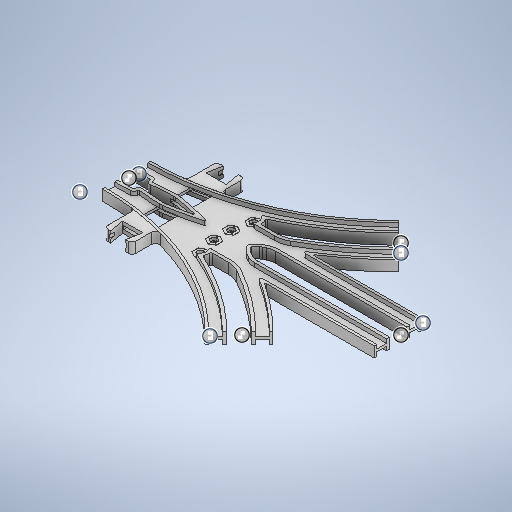
# Autodesk Inventor part: RR_SingleTurnout-all
Saved by Autodesk Inventor 2025.1 (Build 291241000, 241)
## iProperties
Created: 2025-03-05
Part Number: RR_SingleTurnout-all
Material: 一般
Document SubType Name: Modeling
Designer: kumagai
Density: 1 g/cm^3
Appearance: 既定
d0: 244.000 mm
d1: 10.000 mm
d2: 215.000 mm
d3: 5.000 mm
d4: 38.000 mm
d5: 18.600 mm
d6: 2.000 mm
d7: 2.400 mm
d8: 215.000 mm
d9: 45.00 deg
d11: 15.000 mm
d12: 15.000 mm
d13: 2.000 mm
d14: 0.00 deg
d15: 8.400 mm
d16: 0.00 deg
d17: 0.500 mm
d18: 1.000 mm
d19: 20.000 mm
d20: 15.000 mm
d23: 2.500 mm
d30: 5.000 mm
d32: 4.000 mm
d33: 3.000 mm
d34: 4.500 mm
d35: 2.400 mm
d36: 4.000 mm
d37: 1.000 mm
d38: 5.000 mm
d39: 19.000 mm
d41: 0.000 mm
d42: 0.000 mm
d43: 0.000 mm
d44: 0.000 mm
d45: 0.000 mm
d46: 0.000 mm
d47: 0.000 mm
d48: 0.000 mm
d49: 0.000 mm
d51: 5.000 mm
d52: 10.200 mm
d53: 0.300 mm
d55: 2.400 mm
d56: 10.000 mm
d57: 8.000 mm
d58: 0.300 mm
d59: 2.000 mm
d60: 5.000 mm
d62: 2.400 mm
d63: 1.200 mm
d65: 1.200 mm
d66: 42.200 mm
d67: 45.800 mm
TurnoutRadius: 215.000 mm
d40: 19.000 mm
d50: 10.200 mm
PrinterOffset: 0.000 mm
StraightLength: 215.000 mm
RailWidth: 38.000 mm
OuterWall: 2.000 mm
InnerWall: 2.400 mm
InsideWidth: 18.600 mm
RailHeight: 8.400 mm
RailDepth: 3.200 mm
ConnectorLength: 15.000 mm
JointMW1: 13.000 mm
JointMW2: 9.400 mm
JointMH: 9.000 mm
JointFW1: 13.300 mm
JointFW2: 9.600 mm
JointFH: 9.500 mm
DoubleWidth: 60.000 mm
ViaductHeight: 66.000 mm
SupportGap: 0.200 mm
SupportRib: 0.650 mm
JointRadius: 12.000 mm
JointRSLength: 15.000 mm
JointRSTP: 3.000 mm
RailThick: 2.000 mm
d100: 34.048 mm
d126: 0.081 mm
d174: -0.352 mm
d175: 0.482 mm
d178: 0.336 mm
d179: 0.374 mm
Author: kumagai
Autodesk Inventor part; units mm, degrees
ref_plane "YZ Plane" through (0, 0, 0) normal (1, 0, 0) x (0, 1, 0)
sketch "MainSketch" plane through (0, 0, 0) normal (0, 1, 0) x (-1, 0, 0)
  line L0 (0, -344.2613) -> (0, 286.2613) projected
  line L1 (-272.9287, 0) -> (62.5724, 0) projected
  line L2 (14.6437, -29) -> (-5, -29)
  line L3 (-5, -49.5106) -> (-5, -5.6416)
  line L4 (-5, -48) -> (0, -48)
  line L5 (-5, -10) -> (0, -10)
  line L6 (-5, -38.3) -> (0, -38.3)
  line L7 (-5, -19.7) -> (0, -19.7)
  line L8 (-5, -46) -> (0, -46)
  line L9 (-5, -35.9) -> (0, -35.9)
  line L10 (-5, -22.1) -> (0, -22.1)
  line L11 (-5, -12) -> (0, -12)
  line L12 (-10, -10) -> (-10, -29)
  line L13 (-225, -48) -> (-225, -29)
  line L14 (-120.9077, -19.7) -> (-225, -19.7)
  arc A0 (-10, -48) -> (-148.5929, -105.4071) centre (-10, -244) ccw
  arc A1 (-10, -46) -> (-150.0071, -103.9929) centre (-10, -244) ccw
  line L15 (-143.2215, -110.7785) -> (-189.5102, -64.4898)
  line L16 (-210, -35.9) -> (-210, -29)
  line L17 (-146.1596, -86.6272) -> (-155.9415, -76.8453)
  arc A2 (-133.8847, -47.8455) -> (-174.0488, -79.9512) centre (-10, -244) ccw
  arc A3 (-139.2229, -48.9168) -> (-175.463, -78.537) centre (-10, -244) ccw
  line L18 (-139.499, -48) -> (-225, -48)
  line L19 (-134.4186, -46) -> (-225, -46)
  arc A4 (-118.9103, -50.6657) -> (-166.907, -87.093) centre (-10, -244) ccw
  arc A5 (-120.0882, -48.5746) -> (-168.6041, -85.3959) centre (-10, -244) ccw
  line L20 (-94.2219, -46) -> (-110.2721, -46)
  arc A6 (-111.9271, -35.5897) -> (-114.1724, -36.7028) centre (-10, -244) ccw
  line L21 (-120.9077, -35.9) -> (-225, -35.9)
  line L22 (-120.9077, -38.3) -> (-225, -38.3)
  arc A7 (-133.8847, -47.8455) -> (-134.4186, -46) centre (-134.4186, -47) ccw
  arc A8 (-139.2229, -48.9168) -> (-139.499, -48) centre (-139.499, -48.5) ccw
  arc A9 (-110.2721, -48.4) -> (-118.9103, -50.6657) centre (-110.2721, -66) ccw
  arc A10 (-110.2721, -46) -> (-120.0882, -48.5746) centre (-110.2721, -66) ccw
  arc A11 (-120.9077, -38.3) -> (-114.1724, -36.7028) centre (-120.9077, -23.3) ccw
  arc A12 (-120.9077, -35.9) -> (-115.25, -34.5584) centre (-120.9077, -23.3) ccw
  arc A13 (-143.5264, -51.2283) -> (-148.5252, -54.7884) centre (-10, -244) ccw
  arc A14 (-112.9815, -33.4337) -> (-115.25, -34.5584) centre (-10, -244) ccw
  line L23 (-120.9077, -22.1) -> (-225, -22.1)
  circle A15 centre (-86.125, -22.2) radius 2.5
  arc A16 (-96.415, -52.9331) -> (-105.3417, -57.2273) centre (-10, -244) ccw
  arc A17 (-96.4922, -49.4759) -> (-95.7188, -53.2122) centre (-89.6121, -50) ccw
  arc A18 (-93.3838, -47.5455) -> (-92.1285, -53.7307) centre (-89.6121, -50) ccw
  arc A19 (-96.1897, -54.5879) -> (-157.1489, -96.8511) centre (-10, -244) ccw
  line L24 (-97.4893, -48.4) -> (-110.2721, -48.4)
  arc A20 (-92.2877, -55.4762) -> (-155.4519, -98.5481) centre (-10, -244) ccw
  arc A21 (-92.2877, -55.4762) -> (-92.1285, -53.7307) centre (-92.6877, -54.5597) ccw
  arc A22 (-93.3838, -47.5455) -> (-94.2219, -46) centre (-94.2219, -47) ccw
  arc A23 (-96.1897, -54.5879) -> (-95.7188, -53.2122) centre (-96.6039, -53.6777) ccw
  arc A24 (-96.4922, -49.4759) -> (-97.4893, -48.4) centre (-97.4893, -49.4) ccw
  circle A25 centre (-89.6121, -50) radius 2.5
  line L25 (-42.4799, -17.7596) -> (-25.8571, -19.9879)
  arc A26 (-25.9153, -20.5847) -> (-85.6348, -24.6515) centre (-40.1446, -252.1479) ccw
  arc A27 (-85.7928, -19.7222) -> (-85.6348, -24.6515) centre (-86.125, -22.2) ccw
  arc A28 (-25.9153, -20.5847) -> (-25.8571, -19.9879) centre (-25.8969, -20.2853) ccw
  arc A29 (-42.4799, -17.7596) -> (-76.3848, -20.5664) centre (-40.1446, -252.1479) ccw
  line L26 (-85.7928, -19.7222) -> (-79.2595, -20.598)
  arc A30 (-79.2595, -20.598) -> (-76.3848, -20.5664) centre (-77.9308, -10.6866) ccw
  circle A31 centre (-89.6121, -50) radius 4
  line L27 (-89.754, -46.0025) -> (-25.5965, -43.7259)
  arc A32 (-25.552, -44.3238) -> (-40.8225, -46.6677) centre (-3.1703, -241.0547) ccw
  arc A33 (-25.552, -44.3238) -> (-25.5965, -43.7259) centre (-25.5859, -44.0257) ccw
  arc A34 (-74.4895, -48.1141) -> (-87.9633, -53.6443) centre (-3.1703, -241.0547) ccw
  line L28 (-72.9332, -47.8071) -> (-40.8225, -46.6677)
  arc A35 (-72.9332, -47.8071) -> (-74.4895, -48.1141) centre (-72.7559, -52.804) ccw
  arc A36 (-44.0479, -18.9806) -> (-84.6326, -23.2308) centre (-40.1446, -252.1479) ccw
  arc A37 (-27.9859, -39.0878) -> (-44.4613, -41.2072) centre (-10, -244) ccw
  line L29 (-31.1334, -19.7) -> (-47.6548, -19.7)
  arc A38 (-10, -22.1) -> (-22.0271, -22.4262) centre (-10, -244) ccw
  arc A39 (-44.7432, -24.8368) -> (-62.9678, -28.5145) centre (-10, -244) ccw
  arc A40 (-10, -19.7) -> (-22.1572, -20.0297) centre (-10, -244) ccw
  arc A41 (-45.119, -22.4664) -> (-72.2793, -28.5197) centre (-10, -244) ccw
  arc A42 (-25.457, -23.6967) -> (-43.178, -22.3501) centre (-51.8841, -254.1867) ccw
  line L30 (-24.9, -22.9254) -> (-24.9, -23.2)
  arc A43 (-25.457, -23.6967) -> (-24.9, -23.2) centre (-25.4, -23.2) ccw
  arc A44 (-22.1572, -20.0297) -> (-24.9, -22.9254) centre (-22, -22.9254) ccw
  arc A45 (-43.178, -22.3501) -> (-45.119, -22.4664) centre (-43.5532, -32.343) ccw
  arc A46 (-25.7303, -26.0811) -> (-43.268, -24.7484) centre (-51.8841, -254.1867) ccw
  arc A47 (-22.0271, -22.4262) -> (-22.5, -22.9254) centre (-22, -22.9254) ccw
  line L31 (-22.5, -22.9254) -> (-22.5, -23.2)
  arc A48 (-25.7303, -26.0811) -> (-22.5, -23.2) centre (-25.4, -23.2) ccw
  arc A49 (-43.268, -24.7484) -> (-44.7432, -24.8368) centre (-43.5532, -32.343) ccw
  line L32 (-55.2, -53.283) -> (-55.2, -10)
  line L33 (-40.8, -50.4351) -> (-40.8, -10)
  line L34 (-48, 3.552) -> (-48, 5.2256)
  line L35 (-59, -61.5) -> (-37, -61.5)
  line L36 (-40.8, -10) -> (-40.8, -7.4996)
  line L37 (-55.2, -10) -> (-55.2, -7.4996)
  line L38 (-48, -61.9179) -> (-48, -64.1825)
  line L39 (-37, -61.5) -> (-37, -70.5)
  line L40 (-40, -73.5) -> (-42, -73.5)
  line L41 (-42, -73.5) -> (-40, -62)
  line L42 (-40, -62) -> (-56, -62)
  line L43 (-56, -62) -> (-54, -73.5)
  line L44 (-54, -73.5) -> (-56, -73.5)
  line L45 (-59, -70.5) -> (-59, -58.1371)
  arc A50 (-40, -73.5) -> (-37, -70.5) centre (-40, -70.5) ccw
  arc A51 (-59, -70.5) -> (-56, -73.5) centre (-56, -70.5) ccw
  line L46 (-37, -61.5) -> (-37, -49.8686)
  line L47 (-40.8, -50.4351) -> (-40.8, -62)
  line L48 (-55.2, -53.283) -> (-55.2, -62)
  arc A52 (-34.3731, -49.5213) -> (-37, -52.498) centre (-34, -52.498) ccw
  arc A53 (-59, -58.1371) -> (-62.8083, -55.2481) centre (-62, -58.1371) ccw
  line L49 (-10, -29) -> (-225, -29)
  arc A54 (-151.7465, 120.5538) -> (-11.4945, 29.8813) centre (-10, 186) ccw
  arc A55 (-22.0271, -35.5738) -> (-10, -35.9) centre (-10, 186) ccw
  arc A56 (-62.9678, -29.4855) -> (-44.7432, -33.1632) centre (-10, 186) ccw
  arc A57 (-22.1572, -37.9703) -> (-10, -38.3) centre (-10, 186) ccw
  arc A58 (-72.2793, -29.4803) -> (-45.119, -35.5336) centre (-10, 186) ccw
  arc A59 (-43.178, -35.6499) -> (-25.457, -34.3033) centre (-51.8841, 196.1867) ccw
  arc A60 (-43.268, -33.2516) -> (-25.7303, -31.9189) centre (-51.8841, 196.1867) ccw
  arc A61 (-45.119, -35.5336) -> (-43.178, -35.6499) centre (-43.5532, -25.657) ccw
  arc A62 (-44.7432, -33.1632) -> (-43.268, -33.2516) centre (-43.5532, -25.657) ccw
  line L50 (-24.9, -35.0746) -> (-24.9, -34.8)
  arc A63 (-24.9, -35.0746) -> (-22.1572, -37.9703) centre (-22, -35.0746) ccw
  arc A64 (-22.5, -35.0746) -> (-22.0271, -35.5738) centre (-22, -35.0746) ccw
  line L51 (-22.5, -35.0746) -> (-22.5, -34.8)
  arc A65 (-24.9, -34.8) -> (-25.457, -34.3033) centre (-25.4, -34.8) ccw
  arc A66 (-22.5, -34.8) -> (-25.7303, -31.9189) centre (-25.4, -34.8) ccw
  arc A67 (-62.9678, -28.5145) -> (-63.3485, -29) centre (-62.8485, -29) ccw
  arc A68 (-72.2793, -28.5197) -> (-72.6405, -29) centre (-72.1405, -29) ccw
  arc A69 (-108.1902, -15.666) -> (-89.3785, -23.7845) centre (-10, 186) ccw
  arc A70 (-91.0057, 5.3288) -> (-16.6975, -11.8867) centre (-10, 186) ccw
  arc A71 (-122.8924, 131.193) -> (-43.8763, 65.1658) centre (-10, 186) ccw
  arc A72 (-148.5252, -3.2116) -> (-143.5264, -6.7717) centre (-10, 186) ccw
  circle A73 centre (-86.125, -35.8) radius 2.5
  arc A74 (-85.7286, -33.3316) -> (-25.8975, -35.1189) centre (-48.9436, 195.7336) ccw
  line L52 (-25.8166, -35.7131) -> (-42.3424, -38.5735)
  arc A75 (-25.8166, -35.7131) -> (-25.8975, -35.1189) centre (-25.8677, -35.4174) ccw
  line L53 (-85.6986, -38.2634) -> (-79.2034, -37.1391)
  arc A76 (-76.3296, -37.0611) -> (-79.2034, -37.1391) centre (-77.4979, -46.9926) ccw
  arc A77 (-76.3296, -37.0611) -> (-42.3424, -38.5735) centre (-48.9436, 195.7336) ccw
  arc A78 (-49.1227, -37.4664) -> (-46.0444, -37.4484) centre (-48.9436, 195.7336) ccw
  line L54 (-86.4807, -38.2746) -> (-94.1197, -37.1765)
  arc A79 (-94.2268, -36.2144) -> (-94.1197, -37.1765) centre (-94.0486, -36.6816) ccw
  line L55 (-87.0159, -33.4641) -> (-94.2268, -36.2144)
  line L56 (-76.4926, -34.8148) -> (-77.6457, -34.6296)
  arc A80 (-96.055, -36.8647) -> (-107.6082, -42.0517) centre (-10, -244) ccw
  circle A81 centre (-89.6121, -8) radius 4
  line L57 (-89.6178, -12) -> (-25.42, -12.0915)
  arc A82 (-88.0883, -4.3016) -> (-74.4341, -9.37) centre (-9.7235, 185.8863) ccw
  arc A83 (-74.4341, -9.37) -> (-72.8683, -9.6239) centre (-72.8611, -4.6239) ccw
  line L58 (-72.8683, -9.6239) -> (-40.7373, -9.6697)
  arc A84 (-40.7373, -9.6697) -> (-25.3959, -11.4925) centre (-9.7235, 185.8863) ccw
  arc A85 (-25.42, -12.0915) -> (-25.3959, -11.4925) centre (-25.4196, -11.7915) ccw
  line L59 (-41.4, -73.5) -> (-41.4, -70.05)
  line L60 (-54.6, -73.5) -> (-54.6, -70.05)
  line L61 (-21.7393, -64.7371) -> (-21.7393, -55.7371)
  line L62 (-51.6, 5.7033) -> (-51.6, 3.6437)
  line L63 (-44.4, 6.6538) -> (-44.4, 3.6437)
  line L64 (-44.4, -63.9796) -> (-44.4, -61.3243)
  line L65 (-51.6, -63.5159) -> (-51.6, -61.3243)
  arc A86 (-106.8215, -31.0506) -> (-105.9722, -29) centre (-108.8722, -29) ccw
  arc A87 (-111.9271, -35.5897) -> (-109.9456, -34.1747) centre (-115.1782, -28.9421) ccw
  line L66 (-109.9456, -34.1747) -> (-106.8215, -31.0506)
  arc A88 (-112.9815, -33.4337) -> (-111.6427, -32.4776) centre (-115.1782, -28.9421) ccw
  arc A89 (-108.5186, -29.3536) -> (-108.3722, -29) centre (-108.8722, -29) ccw
  line L67 (-111.6427, -32.4776) -> (-108.5186, -29.3536)
  arc A90 (-63.3485, -29) -> (-62.9678, -29.4855) centre (-62.8485, -29) ccw
  arc A91 (-72.6405, -29) -> (-72.2793, -29.4803) centre (-72.1405, -29) ccw
  line L68 (-210, -29) -> (-210, -22.1)
  line L69 (-225, -29) -> (-225, -10)
  line L70 (-10, -29) -> (-10, -48)
  line L71 (-22.0231, -12) -> (-39.3668, -12)
  line L72 (-157.1489, -96.8511) -> (-146.5423, -86.2445)
  point P0 (0, 0)
  point P1 (-90.8602, -19.7)
  point P2 (-94.9346, -22.1)
  point P3 (-96.3241, -48.4)
  point P4 (-87.5506, -46)
  point P5 (-162.028, -91.972)
  point P6 (-44.0258, -45.5806)
  point P7 (-40.8, -24.8544)
  point P8 (-55.2, -26.7523)
  point P9 (-55.2, -44.7764)
  point P10 (-40.8, -44.2654)
  point P11 (-48, -2.9806)
  point P12 (-48, -61.5806)
  point P13 (-37, -73.5)
  point P14 (-59, -73.5)
  point P15 (-59, -54.2238)
  point P16 (-10, -35.9)
  point P17 (-10, -38.3)
  point P18 (-51.2642, -37.4549)
  point P19 (-51.1178, -10.8549)
  point P20 (-103.3722, -29)
  point P21 (-55.2, -31.2477)
  point P22 (-40.8, -33.1456)
  point P23 (-10, -38.3)
  point P24 (-111.9271, -35.5897)
  point P25 (-10, -35.9)
  point P26 (-112.9815, -33.4337)
  point P27 (-40.8, -61.5)
  point P28 (-53.9886, -53)
  point P29 (-48, -53.4549)
  point P30 (-55.2, -61.5)
  dimension "d3" = 5
  dimension "DoubleWidth" = 60
  dimension "d0" = 244
  dimension "d1" = 10
  dimension "d2" = 215
  dimension "d4" = 38
  dimension "d5" = 18.6
  dimension "d6" = 2
  dimension "d7" = 2.4
  dimension "d8" = 215
  dimension "d9" = 45
  dimension "d11" = 15
  dimension "d12" = 15
  dimension "d17" = 0.5
  dimension "d18" = 1
  dimension "d19" = 20
  dimension "d20" = 15
  dimension "d23" = 2.5
  dimension "d30" = 5
  dimension "d32" = 4
  dimension "d34" = 4.5
  dimension "d35" = 2.4
  dimension "d36" = 4
  dimension "d37" = 1
  dimension "d38" = 5
  dimension "d39" = 19
  dimension "d40" = 19
  dimension "d51" = 5
  dimension "d52" = 10.2
  dimension "d53" = 0.3
  dimension "d55" = 2.4
  dimension "d56" = 10
  dimension "d57" = 8
  dimension "d58" = 0.3
  dimension "d60" = 5
  dimension "d62" = 2.4
  dimension "d63" = 1.2
  dimension "d65" = 1.2
  dimension "d66" = 42.2
  dimension "d67" = 45.8
  dimension "d76" = 0.5
  dimension "d78" = 12
  dimension "d79" = 10
  dimension "d80" = 3.5
  dimension "d81" = 0.5
  dimension "d100" = 34.0479
  dimension "d101" = 26.6
  dimension "d102" = 38
  dimension "d103" = 7.2
  dimension "d104" = 7.2
  dimension "d123" = 16
  dimension "d124" = 16
  dimension "d125" = 32.5
  dimension "d126" = 0.0806
  dimension "d135" = 22
  dimension "d136" = 0.5
  dimension "d137" = 16
  dimension "d138" = 12
  dimension "d139" = 12
  dimension "d140" = 3
  dimension "d145" = 3
  dimension "d147" = 0.5
  dimension "d149" = 10.2
  dimension "d150" = 0.3
  dimension "d151" = 1.2
  dimension "d152" = 2.4
  constraints: 196 point on circle, 137 end point, 101 tangent, 92 centre point, 41 coincident, 40 point on line, 32 equal radius, 26 vertical alignment, 15 collinear, 11 horizontal, 9 parallel, 5 symmetric about line, 5 vertical, 3 perpendicular, 50 other
  measures "d0" distance from line of L1 point (-10, -244)
  measures "d2" distance from line of L2 point (-10, -244)
  measures "d4" distance between parallel lines of L5 L4
  measures "d5" distance between parallel lines of L7 L6
  measures "d6" distance between parallel lines of L8 L4
  measures "d7" distance between parallel lines of L9 L6
  measures "d8" distance between parallel lines of L13 L12
  measures "d11" distance between parallel lines of L16 L13
  measures "d17" radius of A8
  measures "d18" radius of A7
  measures "d19" radius of A10
  measures "d20" radius of A11
  measures "d23" distance from line of point (-86.125, -22.2) L14
  measures "d30" diameter of A15
  measures "d32" distance from line of L20 point (-89.612, -50)
  measures "d34" radius of A18
  measures "d35" radial gap between concentric circles of A17 A18
  measures "d36" radial gap between concentric circles of A16 A20
  measures "d37" radius of A21
  measures "d38" diameter of A25
  measures "d39" distance of point (-162.028, -91.972) A0.end
  measures "d40" distance of A3.end point (-162.028, -91.972)
  measures "d51" diameter of A27
  measures "d52" distance from line of point (-86.125, -22.2) L25
  measures "d53" radius of A28
  measures "d55" radial gap between concentric circles of A29 A26
  measures "d56" radius of A30
  measures "d57" diameter of A31
  measures "d58" radius of A33
  measures "d60" radius of A35
  measures "d62" distance between parallel lines of L27 L28
  measures "d63" distance from line of point (-44.026, -45.581) L27
  measures "d65" radial gap between concentric circles of A26 A36
  measures "d66" distance of point (-86.125, -22.2) A36.start
  measures "d67" distance of point (-89.612, -50) point (-44.026, -45.581)
  measures "d76" radius of A43
  measures "d78" distance from line of L12 A44.centre
  measures "d79" radius of A45
  measures "d80" vertical distance of A40.start A43.centre
  measures "d81" radius of A47
  measures "d100" distance from line of L12 A36.start
  measures "d101" distance of A36.start point (-44.026, -45.581)
  measures "d102" distance between parallel lines of L12 L34
  measures "d103" distance between parallel lines of L33 L34
  measures "d104" distance between parallel lines of L32 L34
  measures "d123" vertical distance of point (-48, -2.981) A36.start
  measures "d124" vertical distance of point (-48, -61.581) point (-44.026, -45.581)
  measures "d125" distance between parallel lines of L2 L35
  measures "d126" distance from line of L35 point (-48, -61.581)
  measures "d135" distance between parallel lines of L45 L39
  measures "d136" distance between parallel lines of L35 L42
  measures "d137" distance of L42.end L41.end
  measures "d138" distance between parallel lines of L35 L40
  measures "d139" distance of L43.end L40.end
  measures "d140" radius of A50
  measures "d145" radius of A52
  measures "d147" radius of A67
  measures "d149" distance from line of A73.centre L52
  measures "d150" radius of A75
  measures "d151" radial gap between concentric circles of A74 A78
  measures "d152" radial gap between concentric circles of A74 A77
extrude "BodyPlate" add sketch "MainSketch" along normal mid plane 2 contours L70 A1 L33 A32 A33 L27 L52 A75 A74 A59 A65 L50 A63 A57 | L33 A74 L32 A58 A61 A59 | A74 A75 L52 L33 | L33 L52 A77 L32 A74 | L32 A74 A73 L55 A79 L54 L53 A76 A77 L27 A31 A34 A35 L28 A1 L15 A20 A21 A18 A22 L20 A10 A5 A2 A7 L19 L13 L22 A11 A6 A87 L66 A86 L49 A91 A58 | A1 L32 L28 A32 L33 | L33 L27 L32 A77 L52 | L32 A77 A76 L53 A73 A74 | L33 L27 A33 A32 | A32 L28 L32 L27 L33 | L28 A35 A34 A31 L27 L32 | A73 L54 A79 L55 | A31
extrude "BodyWall" add sketch "MainSketch" along normal mid plane 8.4 contours L70 A57 A63 L50 A65 A59 L33 A60 A66 L51 A64 A55 | L33 A59 A61 A58 L32 A56 A62 A60 | L32 A58 A91 L49 A90 A56 | L70 A0 L33 A1 | L33 A0 L32 A1 | A86 L66 A87 A6 A11 L22 L13 L21 A12 A14 A88 L67 A89 L49 | L32 A0 L15 A1 | L15 A19 A23 A17 A24 L24 A9 A4 A5 A10 L20 A22 A18 A21 A20 | L19 A7 A2 L15 A3 A8 L18 L13
extrude "SlideChannel" cut sketch "MainSketch" along normal blind 1.4 and the other way blind 1.2 contours L49 L32 A39 A49 A46 L33 | L33 A60 A62 A56 L32 L49 | L33 A59 A61 A58 L32 A56 A62 A60 | L49 A67 A39 L32 | L32 A56 A90 L49 | L33 A74 L32 A58 A61 A59 | L33 L52 A77 L32 A74 | L33 A0 L32 A1 | A1 L32 L28 A32 L33 | L33 L27 L32 A77 L52 | L47 L35 L48 A0 | A32 L28 L32 L27 L33 | L47 L42 L64 L35 | L35 L39 A50 L40 L59 L41 L42 L47 | L35 L65 L42 L48 | L64 L42 L65 L35 | L59 L40 L41 | L43 L44 L60
sketch "SupportSketch" plane through (0, 0, 0) normal (0, 1, 0) x (-1, 0, 0)
  circle A0 centre (-89.6121, -50) radius 2.5 projected
  circle A1 centre (-86.125, -35.8) radius 2.5
  line L0 (-89.6121, -56) -> (-89.6121, -50)
  line L1 (-89.6121, -44) -> (-84.416, -47)
  line L2 (-84.416, -47) -> (-89.6121, -50)
  line L3 (-89.6121, -50) -> (-84.416, -53)
  line L4 (-84.416, -53) -> (-89.6121, -56)
  line L5 (-86.125, -41.8) -> (-86.125, -35.8)
  line L6 (-86.125, -29.8) -> (-80.9288, -32.8)
  line L7 (-80.9288, -32.8) -> (-86.125, -35.8)
  line L8 (-86.125, -35.8) -> (-80.9288, -38.8)
  line L9 (-80.9288, -38.8) -> (-86.125, -41.8)
  line L10 (-89.6121, -50) -> (-89.6121, -44)
  line L11 (-86.125, -35.8) -> (-86.125, -29.8)
  line L12 (-88.9621, -54.8742) -> (-88.9621, -51.1258)
  line L13 (-88.9621, -51.1258) -> (-85.716, -53)
  line L14 (-85.716, -53) -> (-88.9621, -54.8742)
  line L15 (-88.9621, -48.8742) -> (-85.716, -47)
  line L16 (-85.716, -47) -> (-88.9621, -45.1258)
  line L17 (-88.9621, -45.1258) -> (-88.9621, -48.8742)
  line L18 (-85.475, -40.6742) -> (-85.475, -36.9258)
  line L19 (-85.475, -36.9258) -> (-82.2288, -38.8)
  line L20 (-82.2288, -38.8) -> (-85.475, -40.6742)
  line L21 (-85.475, -34.6742) -> (-82.2288, -32.8)
  line L22 (-82.2288, -32.8) -> (-85.475, -30.9258)
  line L23 (-85.475, -30.9258) -> (-85.475, -34.6742)
  line L24 (-86.125, -35.8) -> (-91.3211, -38.8)
  line L25 (-91.3211, -38.8) -> (-91.3211, -32.8)
  line L26 (-91.3211, -32.8) -> (-86.125, -35.8)
  line L27 (-90.6711, -37.6742) -> (-87.425, -35.8)
  line L28 (-87.425, -35.8) -> (-90.6711, -33.9258)
  line L29 (-90.6711, -33.9258) -> (-90.6711, -37.6742)
  line L30 (-89.6121, -55) -> (-93.9422, -52.5)
  line L31 (-93.9422, -52.5) -> (-93.9422, -47.5)
  line L32 (-93.9422, -47.5) -> (-89.6121, -45)
  line L33 (-89.6121, -45) -> (-85.282, -47.5)
  line L34 (-85.282, -47.5) -> (-85.282, -52.5)
  line L35 (-85.282, -52.5) -> (-89.6121, -55)
  line L36 (-89.6121, -52.85) -> (-92.0803, -51.425)
  line L37 (-92.0803, -51.425) -> (-92.0803, -48.575)
  line L38 (-92.0803, -48.575) -> (-89.6121, -47.15)
  line L39 (-89.6121, -47.15) -> (-87.1439, -48.575)
  line L40 (-87.1439, -48.575) -> (-87.1439, -51.425)
  line L41 (-87.1439, -51.425) -> (-89.6121, -52.85)
  line L42 (-86.125, -40.8) -> (-90.4551, -38.3)
  line L43 (-90.4551, -38.3) -> (-90.4551, -33.3)
  line L44 (-90.4551, -33.3) -> (-86.125, -30.8)
  line L45 (-86.125, -30.8) -> (-81.7948, -33.3)
  line L46 (-81.7948, -33.3) -> (-81.7948, -38.3)
  line L47 (-81.7948, -38.3) -> (-86.125, -40.8)
  line L48 (-86.125, -38.65) -> (-88.5931, -37.225)
  line L49 (-88.5931, -37.225) -> (-88.5931, -34.375)
  line L50 (-88.5931, -34.375) -> (-86.125, -32.95)
  line L51 (-86.125, -32.95) -> (-83.6568, -34.375)
  line L52 (-83.6568, -34.375) -> (-83.6568, -37.225)
  line L53 (-83.6568, -37.225) -> (-86.125, -38.65)
  point P0 (0, 0)
  point P1 (-84.5465, -37.7387)
  point P2 (-85.2353, -38.1363)
  point P3 (-87.0147, -38.1363)
  point P4 (-87.7034, -37.7387)
  point P5 (-88.5931, -36.1976)
  point P6 (-88.5931, -35.4024)
  point P7 (-87.7034, -33.8613)
  point P8 (-87.0147, -33.4637)
  point P9 (-85.2353, -33.4637)
  point P10 (-84.5465, -33.8613)
  point P11 (-83.6568, -35.4024)
  point P12 (-83.6568, -36.1976)
  point P13 (-87.1439, -49.6024)
  point P14 (-87.1439, -50.3976)
  point P15 (-88.0337, -51.9387)
  point P16 (-88.7224, -52.3363)
  point P17 (-90.5018, -52.3363)
  point P18 (-91.1906, -51.9387)
  point P19 (-92.0803, -50.3976)
  point P20 (-92.0803, -49.6024)
  point P21 (-91.1906, -48.0613)
  point P22 (-90.5018, -47.6637)
  point P23 (-88.7224, -47.6637)
  point P24 (-88.0337, -48.0613)
  dimension "d113" = 0.65
  dimension "d114" = 0.65
  dimension "d115" = 0.65
  dimension "d116" = 0.65
  dimension "d117" = 6
  dimension "d187" = 0.65
  dimension "d197" = 2.85
  dimension "d198" = 5
  dimension "d199" = 2.85
  dimension "d200" = 5
  dimension "d201" = 1.8619
  constraints: 108 end point, 13 equal length, 7 coincident, 4 collinear, 4 point on line, 2 vertical, 1 centre point, 1 equal radius, 62 other
  measures "d113" distance between parallel lines of L4 L14
  measures "d114" distance between parallel lines of L1 L16
  measures "d115" distance between parallel lines of L9 L20
  measures "d116" distance between parallel lines of L7 L21
  measures "d117" distance of L3.end L0.start
  measures "d187" distance between parallel lines of L25 L29
  measures "d197" distance of L48.end L49.end
  measures "d198" distance of L42.end L43.end
  measures "d199" distance of L36.end L37.end
  measures "d200" distance of L30.end L31.end
  measures "d201" distance between parallel lines of L30 L36
ref_plane "SupportTopSurface" through (0, -1.4, 0) normal (0, 1, 0) x (-1, 0, 0)
ref_plane "SupportMidSurface" through (0, -2, 0) normal (0, 1, 0) x (-1, 0, 0)
extrude "Ring" add sketch "SupportSketch" along normal mid plane 2.4 contours A0 L40 L2 L34 L3 | L39 L15 L33 L2 | L3 L35 L13 L41 | L39 A0 L17 L33 L15 | L13 L35 L12 L41 A0 | L36 L0 L30 L31 L32 L10 L38 A0 L37 | L41 L12 L35 L0 | L10 L33 L17 L39 | A1 L52 L7 L46 L8 | L51 L21 L45 L7 | L8 L47 L19 L53 | L51 A1 L23 L45 L21 | L19 L47 L18 L53 A1 | L48 L5 L42 L24 A1 | L53 L18 L47 L5 | A1 L50 L26 L44 L11 | L11 L45 L23 L51 | L24 L43 L27 L49 | L49 L28 L43 L26 | L49 L27 L43 L28 A1
ref_plane "BaseSurface" through (0, -4.2, 0) normal (0, 1, 0) x (-1, 0, 0)
extrude "SupportA" add sketch "SupportSketch" along normal up to surface (2.8 mm away) from surface at -4.2 separate body contours L2 L10 A0 L17 L15 | A0 L15 L39 L2 | L39 L15 L33 L2 | L3 L41 L13 A0 | A0 L13 L12 L0 L3 | L3 L35 L13 L41 | L33 L15 L16 L17 L10 L1 L2 | L3 L4 L0 L35 L12 L14 L13 | A0 L12 L41 L0 | L10 L39 L17 A0 | L41 L12 L35 L0 | L10 L33 L17 L39 | L7 L11 A1 L23 L21 | A1 L21 L51 L7 | L51 L21 L45 L7 | L8 L53 L19 A1 | A1 L19 L18 L5 L8 | L8 L47 L19 L53 | L24 A1 L27 L28 L26 | L45 L21 L22 L23 L11 L6 L7 | L8 L9 L5 L47 L18 L20 L19 | A1 L18 L53 L5 | L11 L51 L23 A1 | L24 L49 L27 A1 | A1 L28 L49 L26 | L53 L18 L47 L5 | L11 L45 L23 L51 | L24 L43 L27 L49 | L49 L28 L43 L26 | L24 L25 L26 L43 L28 L29 L27
extrude "SupportB" add sketch "SupportSketch" against normal up to surface (2.2 mm away) from surface at -2 contours L2 L10 A0 L17 L15 | A0 L15 L39 L2 | L39 L15 L33 L2 | L3 L41 L13 A0 | A0 L13 L12 L0 L3 | L3 L35 L13 L41 | L15 L17 A0 L39 | A0 L39 L15 | L33 L15 L16 L17 L10 L1 L2 | L39 A0 L17 L33 L15 | L13 L41 A0 | A0 L41 L12 L13 | L3 L4 L0 L35 L12 L14 L13 | L13 L35 L12 L41 A0 | L39 A0 | A0 L12 L41 L0 | L10 L39 L17 A0 | L33 L17 L16 L15 | A0 L41 | L13 L14 L12 L35 | A0 L17 L39 | A0 L41 L12 | L41 L12 L35 L0 | L10 L33 L17 L39 | L7 L11 A1 L23 L21 | A1 L21 L51 L7 | L51 L21 L45 L7 | L8 L53 L19 A1 | A1 L19 L18 L5 L8 | L8 L47 L19 L53 | L21 L23 A1 L51 | A1 L51 L21 | L24 A1 L27 L28 L26 | L45 L21 L22 L23 L11 L6 L7 | L51 A1 L23 L45 L21 | L19 L53 A1 | A1 L53 L18 L19 | L8 L9 L5 L47 L18 L20 L19 | L19 L47 L18 L53 A1 | L51 A1 | A1 L18 L53 L5 | L11 L51 L23 A1 | L24 L49 L27 A1 | A1 L28 L49 L26 | L45 L23 L22 L21 | A1 L53 | L19 L20 L18 L47 | A1 L23 L51 | A1 L53 L18 | L53 L18 L47 L5 | L11 L45 L23 L51 | L27 L49 A1 | A1 L49 L28 L27 | L24 L43 L27 L49 | A1 L49 L28 | L49 L28 L43 L26 | L49 L27 L43 L28 A1 | A1 L49 | L24 L25 L26 L43 L28 L29 L27 | L27 L29 L28 L43 bodies 2
extrude "SwitchA" add sketch "MainSketch" along normal mid plane 8.4 separate body contours L47 L35 L48 A0 | A0 L46 L35 L47 | A52 L46 A0 | L48 L35 L45 A53 A0 | L47 L42 L64 L35 | L35 L39 A50 L40 L59 L41 L42 L47 | L48 L42 L43 L60 L44 A51 L45 L35 | L35 L65 L42 L48 | L64 L42 L65 L35 | L59 L40 L41 | L43 L44 L60
extrude "SwitchB" cut sketch "MainSketch" along normal blind 1.4 and the other way blind 1.2 contours L47 L35 L48 A0 | L47 L42 L64 L35 | L35 L65 L42 L48 | L64 L42 L65 L35 | L59 L40 L41 | L43 L44 L60 bodies 3
draft "Slope1" angle 30 pull direction (1, 0, 0) fixed plane through (41.4, 0.5333, -72.35) normal (1, 0, 0) faces at (41.6, -1.2, -72.35) (41.6, 1.4, -72.35)
draft "Slope2" angle 30 pull direction (-1, 0, 0) fixed plane through (54.6, 0.5333, -71.2) normal (-1, 0, 0) faces at (54.4, -1.2, -72.35) (54.4, 1.4, -72.35)
ref_plane "MirrorSurface" through (10, 0, -29) normal (0, 0, 1) x (1, 0, 0)
mirror "BodyMirror" about plane through (10, 0, -29) normal (0, 0, 1) bodies 1 3
mirror "SupportMirror" about plane through (10, 0, -29) normal (0, 0, 1) bodies 2
equation "\"d2\" = TurnoutRadius"
equation "\"d4\" = RailWidth"
equation "\"d5\" = InsideWidth"
equation "\"d6\" = OuterWall"
equation "\"d7\" = InnerWall"
equation "\"d8\" = StraightLength"
equation "\"d11\" = JointRSLength"
equation "\"d12\" = JointRSLength"
equation "\"d13\" = RailThick"
equation "\"d15\" = RailHeight"
equation "\"TurnoutRadius\" = StraightLength"
equation "\"RailWidth\" = 38"
equation "\"InsideWidth\" = 18.6"
equation "\"OuterWall\" = 2"
equation "\"InnerWall\" = 2.4"
equation "\"StraightLength\" = 215"
equation "\"JointRSLength\" = 15"
equation "\"RailThick\" = 2"
equation "\"RailHeight\" = 8.4"
